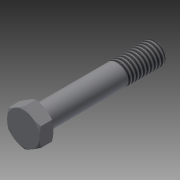
# Autodesk Inventor part: 2.05456-A
Saved by Autodesk Inventor 2014 SP2 (Build 180246200, 246)
## iProperties
Created: 2018-12-09
Part Number: 2.05456-A
Material: Generic
Catalog Web Link: www.cadenas.de
Description: 2 Series Stainless Steel Axle-Capacitiy up to 325 lbs Each
Vendor: COLSONGROUP
Document SubType Name: Modeling
Designer: psadmin
Manufacturer: COLSONGROUP
Mass: 4.77775 g
Surface Area: 21.8235 cm^2
Volume: 4.77775 cm^3
Density: 1 g/cm^3
Appearance: PSOLRGB-175-175-175
Category: PARTsolutions
Company: COLSONGROUP
Title: 2.05456-A
Author: Cadenas PARTsolutions
Comments: Capacitiy up to 325 lbs Each
PSOL_IDENT_0: {$CADENAS_DATA\23d-libs\colsongroup\colson\casters\2_series_stainless_steel\2_series_stainless_steel
PSOL_IDENT_1: _axle.prj},189 {VTYP=3D},{NB=2.05456-A},{LINA=2.05456-A},{NN=2 Series Stainless Steel Axle},{DATE=13
PSOL_IDENT_2: .07.2017 07:15:58},{GEOMDATE=02.03.2017 07:50:00},{VERSION=},{LINEID=10},{WBVAR=MO,D,BR},{WBNUMERIC=
PSOL_IDENT_3: D}  {NB=2.05456-A},{LINA=2.05456-A},{KT=DUMMY},{PN=2.05456},{SER=2 Series Stainless Steel},{MO=TPS},
PSOL_IDENT_4: {MOPN=456},{D=5.00000000},{DALG=3,3.5,4,5},{DPN=05},{BR=},{BRALG= '','None',' BRK1','Top Lock Brake
PSOL_IDENT_5: (BRK1)',' BRK2','Tech Lock Brake (BRK2)',' BRK4','Total Lock Brake (BRK4)' }
NN: 2 Series Stainless Steel Axle
NT: Capacitiy up to 325 lbs Each
NB: 2.05456-A
NBSYN: $PN.-A
LINA: 2.05456-A
PN: 2.05456
SER: 2 Series Stainless Steel
MO: Top Plate Swivel
D: 5
SUPPLIER: COLSONGROUP
ARTICLENO: 2.05456-A
BOMINFO: 2.05456-A
CREATOR: CADENAS GmbH
Autodesk Inventor part; units mm, degrees
sketch "Sketch_2" plane through (0, 0, 0) normal (1, 0, 0) x (0, 1, 0)
  line L0 (0, -52.324) -> (0, 6.096)
  line L1 (0, 6.096) -> (7.112, 6.096)
  line L2 (7.112, 6.096) -> (8.5344, 5.2748)
  line L3 (8.5344, 5.2748) -> (8.5344, 0.8212)
  line L4 (8.5344, 0.8212) -> (7.112, 0)
  line L5 (7.112, 0) -> (4.7625, 0)
  line L6 (4.7625, 0) -> (4.7625, -51.3779)
  line L7 (4.7625, -51.3779) -> (3.8163, -52.324)
  line L8 (3.8163, -52.324) -> (0, -52.324)
  line L9 (0, -52.324) -> (0, 6.096)
  constraints: 20 end point
revolve "Revolution1" add sketch "Sketch_2" angle 360 about axis through (0, 0, -52.324) along (0, 0, -1)
thread "Thread1" size "3/8-16 UNC" class "2A" standard "ANSI Unified Screw Threads" length 16.8338
sketch "Sketch_5" plane through (0, 0, 0) normal (0, 0, 1) x (1, 0, 0)
  circle A0 centre (0, 0) radius 12.7
  line L0 (-7.112, -4.1061) -> (0, -8.2122)
  line L1 (0, -8.2122) -> (7.112, -4.1061)
  line L2 (7.112, -4.1061) -> (7.112, 4.1061)
  line L3 (7.112, 4.1061) -> (0, 8.2122)
  line L4 (0, 8.2122) -> (-7.112, 4.1061)
  line L5 (-7.112, 4.1061) -> (-7.112, -4.1061)
  constraints: 12 end point, 1 centre point
extrude "Extrusion1" cut sketch "Sketch_5" along normal blind 25.4
ref_plane "axle_XY" through (0, 0, 0) normal (0, 0, -1) x (1, 0, 0)
ref_plane "axle_YZ" through (0, 0, 0) normal (1, 0, 0) x (0, -1, 0)
ref_plane "axle_ZX" through (0, 0, 0) normal (0, -1, 0) x (0, 0, -1)
body "Solid1"
